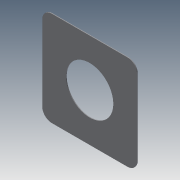
# Autodesk Inventor part: HbSensorTape01
Saved by Autodesk Inventor 2015 SP1 (Build 190203100, 203)
## iProperties
Created: 2016-02-17
Part Number: HbSensorTape01
Material: Generic
Document SubType Name: Modeling
Designer: Yamaura
Density: 1 g/cm^3
Appearance: Default
Author: Yamaura
Autodesk Inventor part; units mm, degrees
ref_plane "YZ Plane" through (0, 0, 0) normal (1, 0, 0) x (0, 1, 0)
ref_plane "XZ Plane" through (0, 0, 0) normal (0, 1, 0) x (-1, 0, 0)
ref_plane "XY Plane" through (0, 0, 0) normal (0, 0, 1) x (1, 0, 0)
sketch "スケッチ1" plane through (0, 0, 0) normal (0, 0, 1) x (1, 0, 0)
  line L0 (-10, 10) -> (10, 10)
  line L1 (10, 10) -> (10, -10)
  line L2 (10, -10) -> (-10, -10)
  line L3 (-10, -10) -> (-10, 10)
  point P0 (0, 0)
  dimension "d0" = 10
  dimension "d1" = 20
  dimension "d2" = 10
  dimension "d3" = 20
  constraints: 8 end point, 2 parallel, 1 horizontal, 1 perpendicular
  measures "d0" distance from line of L3 point (0, 0)
  measures "d1" distance of L0.start L0.end
  measures "d2" distance from line of L0 point (0, 0)
  measures "d3" distance of L0.end L1.end
extrude "押し出し1" add sketch "スケッチ1" along normal blind 0.16
sketch "スケッチ2" plane through (0, 0, 0) normal (0, 0, 1) x (1, 0, 0)
  circle A0 centre (0, 0) radius 5
  dimension "d6" = 10
  constraints: 1 centre point, 1 coincident
  measures "d6" diameter of A0
extrude "押し出し2" cut sketch "スケッチ2" along normal blind 0.16
fillet "フィレット1" radius 2 4 edges at (10, 10, 0.08) (-10, 10, 0.08) (10, -10, 0.08) (-10, -10, 0.08)
